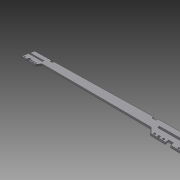
# Autodesk Inventor part: x_axis_chain_holder
Saved by Autodesk Inventor 2014 (Build 180170000, 170)
## iProperties
Created: 2013-12-04
Part Number: x_axis_chain_holder
Material: Generic
Document SubType Name: Modeling
Designer: buben
Density: 1 g/cm^3
Appearance: Default
Author: buben
Autodesk Inventor part; units mm, degrees
ref_plane "YZ Plane" through (0, 0, 0) normal (1, 0, 0) x (0, 1, 0)
ref_plane "XZ Plane" through (0, 0, 0) normal (0, 1, 0) x (-1, 0, 0)
ref_plane "XY Plane" through (0, 0, 0) normal (0, 0, 1) x (1, 0, 0)
sketch "Sketch1" plane through (0, 0, 0) normal (0, 0, 1) x (1, 0, 0)
  line L0 (516, 45) -> (0, 45)
  line L1 (68, 0) -> (78, 15)
  line L2 (78, 15) -> (438, 15)
  line L3 (438, 15) -> (448, 0)
  line L4 (0, 0) -> (68, 0)
  line L5 (448, 0) -> (516, 0)
  line L6 (0, 29) -> (68, 29)
  line L7 (68, 29) -> (68, 23)
  line L8 (68, 23) -> (0, 23)
  line L9 (0, 45) -> (0, 29)
  line L10 (0, 23) -> (0, 0)
  line L11 (516, 29) -> (448, 29)
  line L12 (448, 29) -> (448, 23)
  line L13 (448, 23) -> (516, 23)
  line L14 (516, 0) -> (516, 23)
  line L15 (516, 29) -> (516, 45)
  dimension "d3" = 6
  dimension "d4" = 68
  dimension "d5" = 68
  dimension "d6" = 516
  dimension "d7" = 15
  dimension "d8" = 23
  dimension "d9" = 16
  dimension "d12" = 10
  dimension "d13" = 10
  dimension "d14" = 10
  dimension "d15" = 10
  constraints: 32 end point, 11 perpendicular, 8 parallel, 5 collinear, 2 horizontal
  measures "d3" distance of L6.end L7.end
  measures "d4" distance of L7.end L8.end
  measures "d5" distance of L12.end L13.end
  measures "d6" distance between parallel lines of L14 L10
  measures "d7" distance from line of L1.start L2
  measures "d8" distance of L8.end L4.start
  measures "d9" distance of L0.end L6.start
  measures "d12" distance from line of L7 L1.end
  measures "d13" horizontal distance of L1.start L1.end
  measures "d14" horizontal distance of L2.end L12.end
  measures "d15" horizontal distance of L3.end L2.end
extrude "Extrusion1" add sketch "Sketch1" along normal blind 6
sketch "Sketch2" plane through (0, 0, 6) normal (0, 0, 1) x (1, 0, 0)
  line L0 (0, 0) -> (68, 0) projected
  line L1 (448, 0) -> (516, 0) projected
  line L2 (516, 0) -> (516, 23) projected
  line L3 (516, 29) -> (516, 45) projected
  line L4 (516, 45) -> (0, 45) projected
  line L5 (0, 45) -> (0, 29) projected
  line L6 (0, 23) -> (0, 0) projected
  line L7 (24, 0) -> (35, 0)
  line L8 (35, 0) -> (35, 9)
  line L9 (35, 9) -> (24, 9)
  line L10 (24, 9) -> (24, 0)
  circle A0 centre (42.5, 4.5) radius 2.25
  circle A1 centre (52.5, 3.901) radius 2.75
  circle A2 centre (62.5, 4.5) radius 2.25
  line L11 (492, 0) -> (481, 0)
  line L12 (481, 0) -> (481, 9)
  line L13 (481, 9) -> (492, 9)
  line L14 (492, 9) -> (492, 0)
  circle A3 centre (453.5, 4.5) radius 2.25
  circle A4 centre (463.5, 3.901) radius 2.75
  circle A5 centre (473.5, 4.5) radius 2.25
  line L15 (82.5, 45) -> (92.5, 45)
  line L16 (92.5, 45) -> (92.5, 40)
  line L17 (91.5, 39) -> (83.5, 39)
  line L18 (82.5, 40) -> (82.5, 45)
  line L19 (423.5, 45) -> (433.5, 45)
  line L20 (433.5, 45) -> (433.5, 40)
  line L21 (432.5, 39) -> (424.5, 39)
  line L22 (423.5, 40) -> (423.5, 45)
  arc A6 (82.5, 40) -> (83.5, 39) centre (83.5, 40) ccw
  arc A7 (91.5, 39) -> (92.5, 40) centre (91.5, 40) ccw
  arc A8 (423.5, 40) -> (424.5, 39) centre (424.5, 40) ccw
  arc A9 (432.5, 39) -> (433.5, 40) centre (432.5, 40) ccw
  circle A10 centre (29.5, 3.901) radius 7.5 construction
  point P0 (486.5, 9)
  point P1 (35, 4.5)
  dimension "d16" = 11
  dimension "d18" = 4.5
  dimension "d19" = 5.5
  dimension "d20" = 11
  dimension "d21" = 1
  dimension "d22" = 10
  dimension "d23" = 10
  dimension "d24" = 6
  dimension "d25" = 82.5
  dimension "d26" = 82.5
  dimension "d27" = 24
  dimension "d29" = 23
  dimension "d30" = 24
  dimension "d31" = 10
  dimension "d32" = 10
  dimension "d33" = 10
  dimension "d34" = 10
  dimension "d35" = 9
  dimension "d38" = 15
  dimension "d39" = 23
  constraints: 32 end point, 11 centre point, 10 point on circle, 8 parallel, 8 tangent, 7 equal radius, 6 horizontal alignment, 4 horizontal, 4 perpendicular, 4 point on line, 2 collinear, 2 midpoint
  measures "d16" distance between parallel lines of L8 L10
  measures "d18" diameter of A0
  measures "d19" diameter of A1
  measures "d20" distance between parallel lines of L14 L12
  measures "d21" radius of A6
  measures "d22" distance between parallel lines of L16 L18
  measures "d23" distance between parallel lines of L20 L22
  measures "d24" distance between parallel lines of L4 L17
  measures "d25" distance between parallel lines of L18 L5
  measures "d26" distance between parallel lines of L3 L20
  measures "d27" distance between parallel lines of L6 L10
  measures "d29" horizontal distance of point (486.5, 9) A4.centre
  measures "d30" distance between parallel lines of L2 L14
  measures "d31" horizontal distance of A4.centre A5.centre
  measures "d32" horizontal distance of A4.centre A3.centre
  measures "d33" horizontal distance of A1.centre A0.centre
  measures "d34" horizontal distance of A2.centre A1.centre
  measures "d35" distance of L9.end L7.start
  measures "d38" diameter of A10
  measures "d39" distance of A1.centre A10.centre
extrude "Extrusion2" cut sketch "Sketch2" against normal blind 6
chamfer "Chamfer1" distance 2 angle 45 4 edges at (0, 45, 3) (0, 0, 3) (516, 45, 3) (516, 0, 3)
sketch "Sketch3" plane through (0, 0, 6) normal (0, 0, 1) x (1, 0, 0)
  line L0 (516, 2) -> (516, 23) projected
  line L1 (0, 23) -> (0, 2) projected
  circle A0 centre (52.5, 3.901) radius 2.75 projected
  circle A1 centre (10, 3.901) radius 2
  circle A2 centre (506, 3.901) radius 2
  point P0 (0, 0)
  dimension "d43" = 4
  dimension "d44" = 10
  dimension "d45" = 4
  dimension "d46" = 10
  constraints: 2 centre point, 2 horizontal alignment
  measures "d43" diameter of A1
  measures "d44" distance from line of L1 A1.centre
  measures "d45" diameter of A2
  measures "d46" distance from line of A2.centre L0
extrude "Extrusion3" cut sketch "Sketch3" against normal through all contours A1 | A2
equation "\"d5\" = d4"
equation "\"d20\" = d16"
equation "\"d23\" = d22"
equation "\"d26\" = d25"
equation "\"d30\" = d27"
equation "\"d45\" = d43"
equation "\"d46\" = d44"
body "Solid1"
